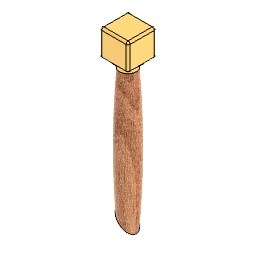
model (Autodesk Fusion 360 design; units mm, degrees)
Autodesk Fusion 360 part; units mm, degrees
sketch "profile" plane through (0, 0, 0) normal (0, 1, 0) x (1, 0, 0)
  line L0 (0, 0) -> (0, 205)
  line L1 (0, 205) -> (12, 205)
  arc A0 (12.2, 0) -> (12, 205) centre (-1332.9051, 101.1878) ccw
  line L2 (0, 0) -> (4.0684, 0)
  line L3 (4.0684, 0) -> (12.2, 0)
  arc A1 (12.2, 0) -> (20.7, -13) centre (24.9269, -0.9574) ccw
  line L4 (20.7, -13) -> (20.7, -50.7)
  line L5 (20.7, -50.7) -> (0, -50.7)
  line L6 (0, -50.7) -> (0, 0)
  line L7 (12, 205) -> (-48, 145)
  line L8 (-48, 145) -> (-48, 205)
  line L9 (-48, 205) -> (12, 205)
  point P0 (16, 102.5038)
  dimension "d1" = 12.2
  dimension "d2" = 12
  dimension "d3" = 205
  dimension "d4" = 16
  dimension "d5" = 20.7
  dimension "d6" = 37.7
  dimension "d7" = 13
  dimension "d10" = 45
  dimension "d11" = 60
  constraint coincident L0.start L2.start
  constraint vertical L0
  constraint horizontal L1
  constraint perpendicular L0 L2
  constraint horizontal L3
  constraint vertical L4
  constraint horizontal L5
  constraint vertical L6
  constraint midpoint A0 P0
  constraint tangent A0 A1
  constraint vertical L8
  constraint horizontal L9
  measures "d1" distance of L0.start A0.start
  measures "d2" distance of L0.end L1.end
  measures "d3" distance of L0.start L0.end
  measures "d4" distance of L0 P0
  measures "d5" distance of L4.end L5.end
  measures "d6" distance of A1.end L4.end
  measures "d7" vertical distance of A0.start A1.end
  measures "d10" angle of L7 L9
  measures "d11" distance of L7.end L8.end
revolve "Revolve1" add sketch "profile" angle 360 about axis through (0, 0, 1.75) along (0, 0, 1) contours L0 A0 L2 L3 L7 | L0 L1 L7 L9 makes body 1
revolve "Revolve2" add sketch "profile" angle 360 about axis through (0, 0, 1.75) along (0, 0, 1) separate body contours L2 L3 A1 L4 L5 L6 makes body 2
extrude "Extrude1" cut sketch "profile" along normal mid plane 160 contours L0 L7 L8 L9 | L0 L1 L7 L9 bodies 1
sketch "top" plane through (0, 0, 50.7) normal (0, 0, 1) x (-1, 0, 0)
  circle A0 centre (0, 0) radius 20.7
  line L0 (-20.7, 20.7) -> (20.7, 20.7)
  line L1 (20.7, 20.7) -> (20.7, -20.7)
  line L2 (20.7, -20.7) -> (-20.7, -20.7)
  line L3 (-20.7, -20.7) -> (-20.7, 20.7)
  line L4 (-20.7, 20.7) -> (20.7, -20.7) construction
  line L5 (20.7, 20.7) -> (-20.7, -20.7) construction
  constraint horizontal L0
  constraint perpendicular L0 L1
  constraint parallel L0 L2
  constraint parallel L1 L3
  constraint coincident L4 A0.centre
  constraint coincident L5 A0.centre
  constraint coincident A0.centre origin
  constraint tangent A0 L2
  constraint tangent A0 L3
extrude "Extrude2" add sketch "top" against normal blind 37.7 bodies 2
fillet "Fillet1" radius 3 4 edges at (-20.7, -20.7, 31.85) (20.7, -20.7, 31.85) (-20.7, 20.7, 31.85) (20.7, 20.7, 31.85) 1 faces at (-6.9, 6.9, 50.7) on bodies 2
fillet "Fillet1" radius 1 4 faces at (-16.6332, -16.6332, 13) (-16.6332, 16.6332, 13) (16.6332, 16.6332, 13) (16.6332, -16.6332, 13) on bodies 2
equation "d1 = ( 24.4 / 2 ) * 1 mm"
equation "d4 = ( 32 / 2 ) * 1 mm"
equation "d5 = ( 41.4 / 2 ) * 1 mm"
equation "d14 = -d6"
